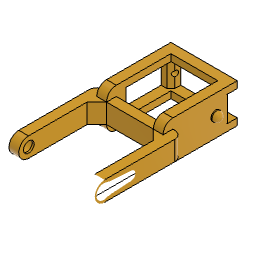
crane assembly v14 (Autodesk Fusion 360 archive; units mm, degrees)
design "link"
Autodesk Fusion 360 part; units mm, degrees
note: some values were not read from the file. Chosen so that the rebuilt part matches the saved one: which bodies a step acts on; which face or edge a step refers to. Set by a fixed rule: which sketch regions a step uses.
sketch "Sketch1" plane through (0, 0, 0) normal (1, 0, 0) x (0, 1, 0)
  line L0 (0, 0) -> (50, 0)
  line L1 (50, 0) -> (50, 10)
  line L2 (50, 10) -> (0, 10)
  line L3 (0, 10) -> (0, 0)
  dimension "d1" = 50
  dimension "d2" = 10
  constraint horizontal L0
  constraint vertical L1
  constraint horizontal L2
  constraint vertical L3
  constraint coincident L0.start L3.end
  measures "d1" distance of L0.start L0.end
  measures "d2" distance of L0.start L2.end
extrude "Extrude1" add sketch "Sketch1" along normal blind 5 makes body 1
sketch "Sketch2" plane through (5, 0, 0) normal (1, 0, 0) x (0, 1, 0)
  line L0 (0, 10) -> (0, 0)
  line L1 (0, 0) -> (50, 0)
  line L2 (50, 0) -> (50, 10)
  line L3 (50, 10) -> (0, 10)
  line L4 (0, 5) -> (4.5, 5) construction
  circle A0 centre (4.5, 5) radius 3.7
  line L5 (4.5, 5) -> (6.5, 5) construction
  line L6 (6.5, 5) -> (6.5, 8.1129)
  line L7 (6.5, 5) -> (6.5, 1.8871)
  line L8 (4.5, 5) -> (18.5, 5) construction
  circle A1 centre (18.5, 5) radius 2.25
  line L9 (18.5, 5) -> (18.5, 7.25) construction
  line L10 (18.5, 5) -> (18.5, 2.75) construction
  line L11 (6.5, 1.8871) -> (18.5, 2.75)
  line L12 (6.5, 8.1129) -> (18.5, 7.25)
  dimension "d5" = 4.5
  dimension "d6" = 7.4
  dimension "d11" = 2
  dimension "d12" = 14
  dimension "d13" = 4.5
  constraint midpoint L0 L4.start
  constraint perpendicular L0 L4
  constraint coincident L4.end A0.centre
  constraint parallel L4 L5
  constraint coincident A0 L6.end
  constraint perpendicular L5 L6
  constraint coincident A0 L7.end
  constraint perpendicular L5 L7
  constraint parallel L5 L8
  constraint coincident L8.end A1.centre
  constraint coincident A1 L9.end
  constraint perpendicular L8 L9
  constraint coincident A1 L10.end
  constraint perpendicular L8 L10
  measures "d5" distance of L4.start L4.end
  measures "d6" diameter of A0
  measures "d11" distance of L4.end L5.end
  measures "d12" distance of L4.end L8.end
  measures "d13" diameter of A1
extrude "Extrude2" cut sketch "Sketch2" against normal blind 5 contours A0 L6 L7 | A0 L6 L7 bodies 1
fillet "Fillet1" radius 5 2 edges at (2.5, 0, 10) (2.5, 0, 0) on bodies 1
extrude "Extrude3" cut sketch "Sketch2" against normal blind 3 contours A0 A1 L11 L12 | A1 bodies 1
fillet "Fillet2" radius 10 2 edges at (3.5, 6.5, 8.1129) (3.5, 6.5, 1.8871) on bodies 1
sketch "Sketch3" plane through (0, 0, 0) normal (-1, 0, 0) x (0, -1, 0)
  circle A0 centre (-4.5, 5) radius 3.7
  arc A1 (-5, 0) -> (-5, 10) centre (-5, 5) ccw
  line L0 (-5, 10) -> (-50, 10)
  line L1 (-50, 10) -> (-50, 0)
  line L2 (-50, 0) -> (-5, 0)
  line L3 (-50, 10) -> (-40, 10) construction
  line L4 (-40, 10) -> (-40, 0) construction
  line L5 (-40, 0) -> (-50, 0) construction
  line L6 (-50, 0) -> (-50, 10) construction
  line L7 (-40, 10) -> (-45, 10)
  line L8 (-45, 10) -> (-45, 0)
  line L9 (-45, 0) -> (-40, 0)
  line L10 (-40, 0) -> (-40, 10)
  dimension "d18" = 10
  dimension "d19" = 5
  constraint horizontal L3
  constraint vertical L4
  constraint horizontal L5
  constraint vertical L6
  constraint coincident L0.end L1.start
  constraint horizontal L7
  constraint vertical L8
  constraint horizontal L9
  constraint vertical L10
  measures "d18" distance of L0.end L3.end
  measures "d19" distance of L3.end L7.end
extrude "Extrude4" add sketch "Sketch3" along normal blind 39 contours L0 L2 L7 L8 L9 L10 bodies 1
sketch "Sketch4" plane through (0, 40, 0) normal (0, -1, 0) x (1, 0, 0)
  line L0 (0, 0) -> (0, 10)
  line L1 (0, 10) -> (-39, 10)
  line L2 (-39, 10) -> (-39, 0)
  line L3 (-39, 0) -> (0, 0)
  line L4 (-39, 10) -> (-34, 10)
  line L5 (-34, 10) -> (-34, 0)
  line L6 (-34, 0) -> (-39, 0)
  line L7 (-39, 0) -> (-39, 10)
  dimension "d22" = 5
  constraint horizontal L4
  constraint vertical L5
  constraint horizontal L6
  constraint vertical L7
  constraint coincident L1.end L2.start
  measures "d22" distance of L1.end L4.end
extrude "Extrude5" add sketch "Sketch4" along normal blind 40 contours L1 L2 L3 L4 L5 L6 L7 bodies 1
sketch "Sketch5" plane through (-34, 0, 0) normal (1, 0, 0) x (0, 1, 0)
  line L0 (40, 0) -> (40, 10)
  line L1 (40, 10) -> (0, 10)
  line L2 (0, 10) -> (0, 0)
  line L3 (0, 0) -> (40, 0)
  line L4 (0, 5) -> (5.175, 5) construction
  circle A0 centre (5.175, 5) radius 2.75
  dimension "d25" = 5.175
  dimension "d26" = 5.5
  constraint midpoint L2 L4.start
  constraint perpendicular L2 L4
  constraint coincident L4.end A0.centre
  measures "d25" distance of L4.start L4.end
  measures "d26" diameter of A0
extrude "Extrude6" cut sketch "Sketch5" against normal blind 3 contours A0 bodies 1
fillet "Fillet3" radius 2 1 edges at (-37, 2.6111, 5.9944) on bodies 1
fillet "Fillet4" radius 5 2 edges at (-36.5, 0, 10) (-36.5, 0, 0) on bodies 1
sketch "Sketch6" plane through (0, 0, 0) normal (0, 0, -1) x (1, 0, 0)
  line L0 (0, -40) -> (-34, -40)
  line L1 (-34, -40) -> (-34, -5)
  line L2 (-34, -5) -> (-39, -5)
  line L3 (-39, -5) -> (-39, -45)
  line L4 (-39, -45) -> (0, -45)
  line L5 (0, -40) -> (5, -40)
  line L6 (5, -40) -> (5, -35)
  line L7 (5, -35) -> (0, -35)
  line L8 (0, -35) -> (0, -40)
  line L9 (0, -45) -> (0, -50)
  line L10 (0, -50) -> (5, -50)
  line L11 (5, -50) -> (5, -5)
  line L12 (5, -5) -> (0, -5)
  line L13 (0, -5) -> (0, -40)
  line L14 (5, -50) -> (0, -50)
  line L15 (0, -50) -> (0, -45)
  line L16 (0, -45) -> (5, -45)
  line L17 (5, -45) -> (5, -50)
  dimension "d35" = 5
  constraint horizontal L5
  constraint vertical L6
  constraint horizontal L7
  constraint vertical L8
  constraint horizontal L14
  constraint vertical L15
  constraint horizontal L16
  constraint vertical L17
  constraint coincident L4.end L9.start
  constraint coincident L10.end L11.start
  measures "d35" distance of L0.start L7.end
extrude "Extrude8" add sketch "Sketch6" along normal blind 5 contours L9 L10 L11 L14 L15 L16 L17 bodies 1
sketch "Sketch7" plane through (0, 0, 10) normal (0, 0, 1) x (-1, 0, 0)
  line L0 (0, -45) -> (39, -45)
  line L1 (39, -45) -> (39, -5)
  line L2 (39, -5) -> (34, -5)
  line L3 (34, -5) -> (34, -40)
  line L4 (34, -40) -> (0, -40)
  line L5 (0, -40) -> (-5, -40)
  line L6 (-5, -40) -> (-5, -35)
  line L7 (-5, -35) -> (0, -35)
  line L8 (0, -35) -> (0, -40)
  line L9 (0, -40) -> (0, -5)
  line L10 (0, -5) -> (-5, -5)
  line L11 (-5, -5) -> (-5, -50)
  line L12 (-5, -50) -> (0, -50)
  line L13 (0, -50) -> (0, -45)
  line L14 (0, -50) -> (-5, -50)
  line L15 (-5, -50) -> (-5, -45)
  line L16 (-5, -45) -> (0, -45)
  line L17 (0, -45) -> (0, -50)
  dimension "d38" = 5
  dimension "d93" = 5
  constraint horizontal L5
  constraint vertical L6
  constraint horizontal L7
  constraint vertical L8
  constraint horizontal L14
  constraint vertical L15
  constraint horizontal L16
  constraint vertical L17
  constraint coincident L12.end L13.start
  measures "d38" distance of L4.end L7.end
  measures "d93" distance of L12.end L0.start
extrude "Extrude9" add sketch "Sketch7" along normal blind 5 contours L11 L12 L13 L14 L15 L16 L17 bodies 1
sketch "Sketch8" plane through (0, 45, 0) normal (0, 1, 0) x (-1, 0, 0)
  line L0 (0, 0) -> (39, 0)
  line L1 (39, 0) -> (39, 10)
  line L2 (39, 10) -> (0, 10)
  line L3 (39, 0) -> (34, 0)
  line L4 (34, 0) -> (34, 15)
  line L5 (34, 15) -> (39, 15)
  line L6 (39, 15) -> (39, 0)
  line L7 (39, 0) -> (34, 0)
  line L8 (34, 0) -> (34, -5)
  line L9 (34, -5) -> (39, -5)
  line L10 (39, -5) -> (39, 0)
  line L11 (0, 10) -> (0, 0)
  dimension "d41" = 5
  dimension "d42" = 15
  dimension "d43" = 5
  dimension "d44" = 5
  constraint horizontal L3
  constraint vertical L4
  constraint horizontal L5
  constraint vertical L6
  constraint coincident L0.end L1.start
  constraint horizontal L7
  constraint vertical L8
  constraint horizontal L9
  constraint vertical L10
  measures "d41" distance of L0.end L3.end
  measures "d42" distance of L0.end L5.end
  measures "d43" distance of L0.end L3.end
  measures "d44" distance of L0.end L9.end
extrude "Extrude10" add sketch "Sketch8" along normal blind 5 contours L0 L1 L2 L3 L4 L6 L7 | L0 L3 L7 L8 L9 L10 | L2 L4 L5 L6 bodies 1
split "Split1" by plane through (0, 45, 10) normal (0, 1, 0) bodies 1 makes body 2 at (-34, 48.3333, 3.3333) makes body 3 at (0, 48.3333, 3.3333)
move_body "Move1" bodies 2 to x (1, 0, 0) y (0, 1, 0) z (0, 0, 1) at (5, 0, 0)
move_body "Move3" bodies 3 to x (1, 0, 0) y (0, 1, 0) z (0, 0, 1) at (-5, 0, 0)
chamfer "Chamfer4" distance 5 angle 45 2 edges at (-34, 40, 5) (0, 40, 5) on bodies 1
combine "Combine1" operation add target body 1 tool bodies 3 2
revolve "Revolve1" add 2 faces at (-3.3333, 45, -1.6667) (-30.6667, 45, -1.6667) angle 360 about axis through (-29, 45, 0) along (1, 0, 0) on bodies 1 bodies 1
revolve "Revolve2" add 2 faces at (-30.6667, 45, 13.3333) (-1.6667, 45, 11.6667) angle 360 about axis through (-5, 45, 10) along (-1, 0, 0) on bodies 1 bodies 1
sketch "Sketch16" plane through (0, 50, 0) normal (0, 1, 0) x (-1, 0, 0)
  line L0 (29, 15) -> (29, -5)
  line L1 (29, -5) -> (34, -5)
  line L2 (34, -5) -> (34, 15)
  line L3 (34, 15) -> (29, 15)
  line L4 (34, -5) -> (29, -5)
  line L5 (29, -5) -> (29, -1.5)
  line L6 (29, -1.5) -> (34, -1.5)
  line L7 (34, -1.5) -> (34, -5)
  line L8 (34, 15) -> (29, 15)
  line L9 (29, 15) -> (29, 11.5)
  line L10 (29, 11.5) -> (34, 11.5)
  line L11 (34, 11.5) -> (34, 15)
  dimension "d96" = 3.5
  dimension "d97" = 3.5
  constraint horizontal L4
  constraint vertical L5
  constraint horizontal L6
  constraint vertical L7
  constraint coincident L1.end L2.start
  constraint horizontal L8
  constraint vertical L9
  constraint horizontal L10
  constraint vertical L11
  constraint coincident L2.end L3.start
  measures "d96" distance of L1.end L6.end
  measures "d97" distance of L2.end L10.end
extrude "Extrude12" add sketch "Sketch16" along normal blind 28 contours L0 L2 L3 L8 L9 L10 L11 | L0 L1 L2 L4 L5 L6 L7 bodies 1
sketch "Sketch17" plane through (0, 0, 11.5) normal (0, 0, -1) x (1, 0, 0)
  line L0 (-29, -50) -> (-34, -50)
  line L1 (-34, -50) -> (-34, -78)
  line L2 (-34, -78) -> (-29, -78)
  line L3 (-29, -78) -> (-29, -50)
  line L4 (-34, -78) -> (-29, -78)
  line L5 (-29, -78) -> (-29, -73)
  line L6 (-29, -73) -> (-34, -73)
  line L7 (-34, -73) -> (-34, -78)
  dimension "d98" = 5
  constraint horizontal L4
  constraint vertical L5
  constraint horizontal L6
  constraint vertical L7
  constraint coincident L1.end L2.start
  measures "d98" distance of L1.end L6.end
extrude "Extrude13" add sketch "Sketch17" along normal blind 13 contours L1 L2 L3 L4 L5 L6 L7 bodies 1
sketch "Sketch12" plane through (-39, 0, 0) normal (-1, 0, 0) x (0, -1, 0)
  line L0 (-73, 5) -> (-75.5, 5) construction
  circle A0 centre (-75.5, 5) radius 1.4
  line L1 (-45, 10) -> (-45, 0)
  line L2 (-45, 0) -> (-5, 0)
  arc A1 (-5, 0) -> (-5, 10) centre (-5, 5) ccw
  line L3 (-5, 10) -> (-45, 10)
  dimension "d64" = 2.5
  dimension "d65" = 2.8
  constraint coincident L0.end A0.centre
  measures "d64" distance of L0.start L0.end
  measures "d65" diameter of A0
extrude "Extrude14" cut sketch "Sketch12" against normal blind 10 contours A0 bodies 1
extrude "Extrude15" add 1 faces at (-1.6667, 50, 1.6667) along direction (0, 1, 0) blind 28 on bodies 1 bodies 1
sketch "Sketch18" plane through (-29, 0, 0) normal (1, 0, 0) x (0, 1, 0)
  circle A0 centre (75.5, 5) radius 1.4
  line L0 (73, -1.5) -> (50, -1.5)
  line L1 (50, -1.5) -> (50, 11.5)
  line L2 (50, 11.5) -> (73, 11.5)
  line L3 (73, 11.5) -> (73, -1.5)
  line L4 (78, -5) -> (78, 15)
  line L5 (78, 15) -> (45, 15)
  arc A1 (45, 15) -> (40, 10) centre (45, 10) ccw
  line L6 (40, 10) -> (45, 10)
  line L7 (45, 10) -> (45, 0)
  line L8 (45, 0) -> (40, 0)
  arc A2 (40, 0) -> (45, -5) centre (45, 0) ccw
  line L9 (45, -5) -> (78, -5)
  line L10 (78, 15) -> (73, 15)
  line L11 (73, 15) -> (73, 11.5)
  line L12 (73, 11.5) -> (78, 11.5)
  line L13 (78, 11.5) -> (78, 15)
  line L14 (78, -5) -> (73, -5)
  line L15 (73, -5) -> (73, -1.5)
  line L16 (73, -1.5) -> (78, -1.5)
  line L17 (78, -1.5) -> (78, -5)
  constraint horizontal L10
  constraint vertical L11
  constraint horizontal L12
  constraint vertical L13
  constraint coincident L2.end L3.start
  constraint coincident L4.end L5.start
  constraint horizontal L14
  constraint vertical L15
  constraint horizontal L16
  constraint vertical L17
  constraint coincident L0.start L3.end
  constraint coincident L4.start L9.end
extrude "Extrude16" add sketch "Sketch18" along normal blind 24 contours L4 L9 L14 L15 L16 L17 | L4 L5 L10 L11 L12 L13 bodies 1
sketch "Sketch14" plane through (0, 0, 0) normal (1, 0, 0) x (0, 1, 0)
  line L0 (78, -5) -> (78, 15)
  line L1 (78, 15) -> (78, 11.5) construction
  line L2 (78, 11.5) -> (73, 11.5)
  line L3 (73, 11.5) -> (73, -1.5)
  line L4 (73, -1.5) -> (78, -1.5)
  line L5 (78, -1.5) -> (78, 11.5)
  line L6 (40, 10) -> (45, 10)
  line L7 (45, 10) -> (45, 0)
  line L8 (45, 0) -> (40, 0)
  line L9 (40, 0) -> (40, 10)
  arc A0 (40, 0) -> (45, -5) centre (45, 0) ccw
  line L10 (45, 10) -> (45, 0)
  line L11 (45, 0) -> (40, 0)
  line L12 (45, -5) -> (78, -5)
  line L13 (78, 15) -> (45, 15)
  arc A1 (45, 15) -> (40, 10) centre (45, 10) ccw
  line L14 (40, 10) -> (45, 10)
  point P0 (40, 0)
  point P1 (40, 0)
  dimension "d75" = 3.5
  dimension "d76" = 5
  dimension "d77" = 13
  dimension "d80" = 5
  dimension "d81" = 10
  constraint coincident L0.end L1.start
  constraint horizontal L2
  constraint vertical L3
  constraint horizontal L4
  constraint vertical L5
  constraint horizontal L6
  constraint vertical L7
  constraint horizontal L8
  constraint vertical L9
  measures "d75" distance of L0.end L1.end
  measures "d76" distance of L1.end L2.end
  measures "d77" distance of L1.end L4.end
  measures "d80" distance of L6.start L6.end
  measures "d81" distance of L6.start P1
extrude "Extrude17" cut sketch "Sketch14" against normal blind 5 contours L0 L2 L3 L4 L5 | L6 L7 L8 L9 L10 L11 L14 bodies 1
sketch "Sketch15" plane through (0, 0, 0) normal (1, 0, 0) x (0, 1, 0)
  line L0 (78, 11.5) -> (78, 15)
  line L1 (73, -1.5) -> (73, 11.5)
  line L2 (73, 11.5) -> (78, 11.5)
  line L3 (73, 5) -> (67, 5) construction
  circle A0 centre (67, 5) radius 2.5
  arc A1 (40, 0) -> (45, -5) centre (45, 0) ccw
  line L4 (78, -1.5) -> (73, -1.5)
  line L5 (78, 15) -> (45, 15)
  arc A2 (45, 15) -> (40, 10) centre (45, 10) ccw
  line L6 (40, 10) -> (45, 10)
  line L7 (45, 10) -> (45, 0)
  line L8 (45, 0) -> (40, 0)
  line L9 (45, -5) -> (78, -5)
  line L10 (78, -5) -> (78, -1.5)
  dimension "d84" = 6
  dimension "d85" = 5
  constraint midpoint L1 L3.start
  constraint coincident L3.end A0.centre
  measures "d84" distance of L3.start L3.end
  measures "d85" diameter of A0
extrude "Extrude18" add sketch "Sketch15" along normal blind 3 contours A0 bodies 1
fillet "Fillet7" radius 2.5 1 edges at (3, 64.6692, 4.096) on bodies 1
chamfer "Chamfer2" distance 5 angle 45 1 edges at (-5, 73, 5) on bodies 1
chamfer "Chamfer5" distance 2 angle 45 1 edges at (-29, 73, 5) on bodies 1
sketch "Sketch19" plane through (-29, 0, 0) normal (1, 0, 0) x (0, 1, 0)
  line L0 (73, 11.5) -> (73, 15)
  line L1 (73, 15) -> (45, 15)
  arc A0 (45, 15) -> (40, 10) centre (45, 10) ccw
  line L2 (40, 10) -> (45, 10)
  line L3 (45, 10) -> (45, 0)
  line L4 (45, 0) -> (40, 0)
  arc A1 (40, 0) -> (45, -5) centre (45, 0) ccw
  line L5 (45, -5) -> (73, -5)
  line L6 (73, -5) -> (73, -1.5)
  line L7 (73, -1.5) -> (50, -1.5)
  line L8 (50, -1.5) -> (50, 11.5)
  line L9 (50, 11.5) -> (73, 11.5)
  line L10 (45, 5) -> (47.5, 5)
  circle A2 centre (47.5, 5) radius 1.4
  dimension "d100" = 2.5
  dimension "d101" = 2.8
  constraint midpoint L3 L10.start
  constraint perpendicular L8 L10
  constraint coincident L10.end A2.centre
  measures "d100" distance of L10.start L10.end
  measures "d101" diameter of A2
extrude "Extrude19" cut sketch "Sketch19" against normal blind 5 contours A2 bodies 1
fillet "Fillet8" radius 4 2 edges at (-39, 45, 5) (5, 45, 5) on bodies 1

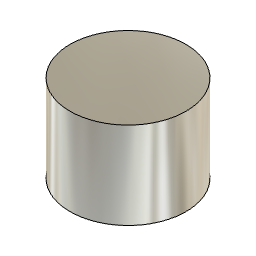
design "electromagnet"
Autodesk Fusion 360 part; units mm, degrees
sketch "Sketch1" plane through (0, 0, 0) normal (0, 0, 1) x (1, 0, 0)
  circle A0 centre (0, 0) radius 10
  dimension "d1" = 20
  constraint coincident A0.centre origin
  measures "d1" diameter of A0
extrude "Extrude1" add sketch "Sketch1" along normal blind 15
sketch "Sketch2" plane through (0, 0, 0) normal (0, 0, -1) x (1, 0, 0)
  circle A0 centre (0, 0) radius 10
  circle A1 centre (0, 0) radius 2
  dimension "d4" = 4
  constraint concentric A0 A1
  measures "d4" diameter of A1
extrude "Extrude2" cut sketch "Sketch2" against normal blind 5 contours A1

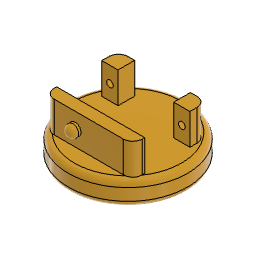
design "first crane stand"
part number: Configuration 1
Autodesk Fusion 360 part; units mm, degrees
sketch "Sketch1" plane through (0, 0, 0) normal (0, 0, 1) x (1, 0, 0)
  circle A0 centre (0, 0) radius 25
  dimension "d1" = 50
  constraint coincident A0.centre origin
  measures "d1" diameter of A0
extrude "Extrude1" add sketch "Sketch1" along normal blind 10
sketch "Sketch2" plane through (0, 0, 0) normal (0, 0, -1) x (1, 0, 0)
  circle A0 centre (0, 0) radius 25
  line L0 (0, 0) -> (0, -10) construction
  circle A1 centre (0, -10) radius 3.5
  line L1 (0, -10) -> (0, -7.737) construction
  line L2 (0, -7.737) -> (-2.67, -7.737) construction
  line L3 (0, -7.737) -> (2.67, -7.737) construction
  line L4 (0, -10) -> (0, 3.98) construction
  circle A2 centre (0, 3.98) radius 2.1005
  line L5 (2.67, -7.737) -> (2.098, 4.0815)
  line L6 (-2.67, -7.737) -> (-2.098, 4.0815)
  dimension "d4" = 10
  dimension "d5" = 7
  dimension "d6" = 2.263
  dimension "d7" = 13.98
  dimension "d8" = 4.201
  constraint coincident A0.centre L0.start
  constraint vertical L0
  constraint coincident L0.end A1.centre
  constraint parallel L0 L1
  constraint coincident A1 L2.end
  constraint perpendicular L0 L2
  constraint coincident A1 L3.end
  constraint perpendicular L1 L3
  constraint parallel L0 L4
  constraint coincident L4.end A2.centre
  constraint coincident A2 L5.end
  constraint tangent A2 L5
  constraint coincident A2 L6.end
  constraint tangent A2 L6
  measures "d4" distance of A0.centre L0.end
  measures "d5" diameter of A1
  measures "d6" distance of L0.end L1.end
  measures "d7" distance of L0.end L4.end
  measures "d8" diameter of A2
extrude "Extrude2" cut sketch "Sketch2" against normal blind 2 contours A1 | A1 A2 L5 L6 | A2
sketch "Sketch14" plane through (0, 0, 10) normal (0, 0, 1) x (-1, 0, 0)
  circle A0 centre (0, 0) radius 25
  line L0 (18.5, 11.5) -> (-18.5, 11.5) construction
  line L1 (-18.5, 11.5) -> (-18.5, -11.5) construction
  line L2 (-18.5, -11.5) -> (18.5, -11.5) construction
  line L3 (18.5, -11.5) -> (18.5, 11.5) construction
  line L4 (18.5, 11.5) -> (-18.5, -11.5) construction
  line L5 (-18.5, 11.5) -> (18.5, -11.5) construction
  line L6 (-18.5, -11.5) -> (-11.7, -11.5)
  line L7 (-11.7, -11.5) -> (-11.7, -7.5)
  line L8 (-11.7, -7.5) -> (-18.5, -7.5)
  line L9 (-18.5, -7.5) -> (-18.5, -11.5)
  line L10 (18.5, -11.5) -> (11.7, -11.5)
  line L11 (11.7, -11.5) -> (11.7, -7.5)
  line L12 (11.7, -7.5) -> (18.5, -7.5)
  line L13 (18.5, -7.5) -> (18.5, -11.5)
  line L14 (18.5, 11.5) -> (-18.5, 11.5)
  line L15 (-18.5, 11.5) -> (-18.5, 16.5)
  line L16 (-18.5, 16.5) -> (18.5, 16.5)
  line L17 (18.5, 16.5) -> (18.5, 11.5)
  dimension "d95" = 37
  dimension "d96" = 23
  dimension "d97" = 6.8
  dimension "d98" = 4
  dimension "d99" = 6.8
  dimension "d100" = 4
  dimension "d101" = 37
  dimension "d102" = 5
  constraint horizontal L0
  constraint perpendicular L0 L1
  constraint parallel L0 L2
  constraint parallel L1 L3
  constraint coincident L4 A0.centre
  constraint coincident L5 A0.centre
  constraint coincident A0.centre origin
  constraint horizontal L6
  constraint vertical L7
  constraint horizontal L8
  constraint vertical L9
  constraint horizontal L10
  constraint vertical L11
  constraint horizontal L12
  constraint vertical L13
  constraint horizontal L14
  constraint vertical L15
  constraint horizontal L16
  constraint vertical L17
  measures "d95" distance of L1.end L2.end
  measures "d96" distance of L0.end L1.end
  measures "d97" distance of L1.end L6.end
  measures "d98" distance of L1.end L8.end
  measures "d99" distance of L2.end L10.end
  measures "d100" distance of L2.end L12.end
  measures "d101" distance of L0.start L0.end
  measures "d102" distance of L0.start L16.end
extrude "Extrude15" add sketch "Sketch14" along normal blind 13 contours L6 L7 L8 L9 | L10 L11 L12 L13 | L14 L15 L16 L17
sketch "Sketch15" plane through (0, 11.5, 0) normal (0, 1, 0) x (-1, 0, 0)
  line L0 (-18.5, 10) -> (-11.7, 10)
  line L1 (-11.7, 10) -> (-11.7, 23)
  line L2 (-11.7, 23) -> (-18.5, 23)
  line L3 (-18.5, 23) -> (-18.5, 10)
  line L4 (-15.1, 10) -> (-15.1, 16.25) construction
  circle A0 centre (-15.1, 16.25) radius 1.4
  dimension "d105" = 6.25
  dimension "d106" = 2.8
  constraint midpoint L0 L4.start
  constraint perpendicular L0 L4
  constraint coincident L4.end A0.centre
  measures "d105" distance of L4.start L4.end
  measures "d106" diameter of A0
sketch "Sketch16" plane through (0, 11.5, 0) normal (0, 1, 0) x (-1, 0, 0)
  line L0 (11.7, 10) -> (18.5, 10)
  line L1 (18.5, 10) -> (18.5, 23)
  line L2 (18.5, 23) -> (11.7, 23)
  line L3 (11.7, 23) -> (11.7, 10)
  line L4 (15.1, 10) -> (15.1, 16.25) construction
  circle A0 centre (15.1, 16.25) radius 1.4
  dimension "d107" = 6.25
  dimension "d108" = 2.8
  constraint midpoint L0 L4.start
  constraint perpendicular L0 L4
  constraint coincident L4.end A0.centre
  measures "d107" distance of L4.start L4.end
  measures "d108" diameter of A0
extrude "Extrude16" cut sketch "Sketch16" sketch "Sketch15" against normal blind 4.475 contours A0 of sketch 2 contours A0
sketch "Sketch17" plane through (0, -16.5, 0) normal (0, -1, 0) x (1, 0, 0)
  line L0 (-18.5, 10) -> (18.5, 10)
  line L1 (18.5, 10) -> (18.5, 23)
  line L2 (18.5, 23) -> (-18.5, 23)
  line L3 (-18.5, 23) -> (-18.5, 10)
  line L4 (-18.5, 10) -> (18.5, 23) construction
  line L5 (18.5, 10) -> (-18.5, 23) construction
  line L6 (0, 16.5) -> (-5.7, 16.5) construction
  circle A0 centre (-5.7, 16.5) radius 2.5
  dimension "d120" = 5.7
  dimension "d121" = 5
  constraint coincident L0.start L3.end
  constraint coincident L1.end L2.start
  constraint coincident L0.end L1.start
  constraint coincident L2.end L3.start
  constraint horizontal L6
  constraint coincident L6.end A0.centre
  measures "d120" distance of L6.start L6.end
  measures "d121" diameter of A0
extrude "Extrude17" add sketch "Sketch17" along normal blind 3.5 contours A0
extrude "Extrude18" add 2 faces at (15.0651, 11.5, 21.2154) (-15.0651, 11.5, 21.2154) along direction (0, 1, 0) blind 3
fillet "Fillet8" radius 2.5 1 faces at (-6.4508, -20, 16.1384)
fillet "Fillet9" radius 4 2 edges at (18.5, -16.5, 16.5) (-18.5, -16.5, 16.5)
fillet "Fillet10" radius 2.5 2 edges at (-23.3082, -9.0404, 10) (-23.3082, -9.0404, 0)
fillet "Fillet11" radius 4 2 edges at (-18.5, 14.5, 16.3945) (18.5, 14.5, 16.3945)
equation "fullServoLength = 32.45 mm"

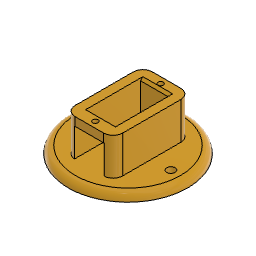
design "crane_base"
Autodesk Fusion 360 part; units mm, degrees
sketch "Sketch1" plane through (0, 0, 0) normal (0, 0, 1) x (1, 0, 0)
  circle A0 centre (0, 0) radius 25
  line L0 (0, 0) -> (-18, 0) construction
  line L1 (0, 0) -> (18, 0) construction
  circle A1 centre (-18, 0) radius 1.75
  circle A2 centre (18, 0) radius 1.75
  dimension "d1" = 50
  dimension "d25" = 18
  dimension "d26" = 18
  dimension "d27" = 3.5
  dimension "d28" = 3.5
  constraint coincident A0.centre L0.start
  constraint horizontal L0
  constraint parallel L0 L1
  constraint coincident L0.end A1.centre
  constraint coincident L1.end A2.centre
  measures "d1" diameter of A0
  measures "d25" distance of A0.centre L0.end
  measures "d26" distance of A0.centre L1.end
  measures "d27" diameter of A1
  measures "d28" diameter of A2
extrude "Extrude1" add sketch "Sketch1" along normal blind 3
sketch "Sketch2" plane through (0, 0, 3) normal (0, 0, 1) x (-1, 0, 0)
  circle A0 centre (0, 0) radius 25
  line L0 (-6.25, 11.5) -> (6.25, 11.5)
  line L1 (6.25, 11.5) -> (6.25, -11.5)
  line L2 (6.25, -11.5) -> (-6.25, -11.5)
  line L3 (-6.25, -11.5) -> (-6.25, 11.5)
  line L4 (-6.25, 11.5) -> (6.25, -11.5) construction
  line L5 (6.25, 11.5) -> (-6.25, -11.5) construction
  line L6 (-10, -16.225) -> (10, -16.225)
  line L7 (10, -16.225) -> (10, 16.225)
  line L8 (10, 16.225) -> (-10, 16.225)
  line L9 (-10, 16.225) -> (-10, -16.225)
  line L10 (-10, -16.225) -> (10, 16.225) construction
  line L11 (10, -16.225) -> (-10, 16.225) construction
  circle A1 centre (-18, 0) radius 1.75
  circle A2 centre (18, 0) radius 1.75
  dimension "d4" = 12.5
  dimension "d5" = 23
  dimension "d6" = 20
  dimension "d7" = 32.45
  constraint horizontal L0
  constraint perpendicular L0 L1
  constraint parallel L0 L2
  constraint parallel L1 L3
  constraint coincident L4 A0.centre
  constraint coincident L5 A0.centre
  constraint coincident A0.centre origin
  constraint horizontal L6
  constraint perpendicular L6 L7
  constraint parallel L6 L8
  constraint parallel L7 L9
  constraint coincident L10 A0.centre
  constraint coincident L11 A0.centre
  measures "d4" distance of L1.end L2.end
  measures "d5" distance of L0.end L1.end
  measures "d6" distance of L7.end L8.end
  measures "d7" distance of L6.end L7.end
extrude "Extrude2" add sketch "Sketch2" along normal blind 15.55 contours L6 L7 L8 L9
sketch "Sketch3" plane through (0, 0, 18.55) normal (0, 0, 1) x (-1, 0, 0)
  line L0 (6.25, -11.5) -> (-6.25, -11.5)
  line L1 (-6.25, -11.5) -> (-6.25, 11.5)
  line L2 (-6.25, 11.5) -> (6.25, 11.5)
  line L3 (6.25, 11.5) -> (6.25, -11.5)
  line L4 (-10, 16.225) -> (-10, -16.225)
  line L5 (-10, -16.225) -> (10, -16.225)
  line L6 (10, -16.225) -> (10, 16.225)
  line L7 (10, 16.225) -> (-10, 16.225)
  line L8 (0, 16.225) -> (0, 13.667) construction
  line L9 (0, -16.225) -> (0, -13.667) construction
  circle A0 centre (0, -13.667) radius 1.1
  circle A1 centre (0, 13.667) radius 1.1
  dimension "d10" = 2.558
  dimension "d11" = 2.558
  dimension "d12" = 2.2
  dimension "d13" = 2.2
  constraint midpoint L7 L8.start
  constraint perpendicular L7 L8
  constraint midpoint L5 L9.start
  constraint perpendicular L5 L9
  constraint coincident L9.end A0.centre
  constraint coincident L8.end A1.centre
  measures "d10" distance of L8.start L8.end
  measures "d11" distance of L9.start L9.end
  measures "d12" diameter of A0
  measures "d13" diameter of A1
extrude "Extrude3" cut sketch "Sketch3" against normal blind 10 contours A0 | A1
sketch "Sketch4" plane through (0, -16.225, 0) normal (0, -1, 0) x (1, 0, 0)
  line L0 (-10, 3) -> (10, 3)
  line L1 (10, 3) -> (10, 18.55)
  line L2 (10, 18.55) -> (-10, 18.55)
  line L3 (-10, 18.55) -> (-10, 3)
  line L4 (0, 3) -> (-6.25, 3) construction
  line L5 (-6.25, 3) -> (6.25, 3)
  line L6 (6.25, 3) -> (6.25, 15)
  line L7 (6.25, 15) -> (-6.25, 15)
  line L8 (-6.25, 15) -> (-6.25, 3)
  dimension "d16" = 6.25
  dimension "d17" = 12.5
  dimension "d18" = 12
  constraint midpoint L0 L4.start
  constraint parallel L0 L4
  constraint horizontal L5
  constraint vertical L6
  constraint horizontal L7
  constraint vertical L8
  measures "d16" distance of L4.start L4.end
  measures "d17" distance of L4.end L5.end
  measures "d18" distance of L4.end L7.end
extrude "Extrude4" cut sketch "Sketch4" against normal blind 4.725 contours L0 L5 L6 L7 L8
fillet "Fillet2" radius 4 4 edges at (10, -16.225, 10.775) (10, 16.225, 10.775) (-10, 16.225, 10.775) (-10, -16.225, 10.775)
fillet "Fillet3" radius 3 1 edges at (-23.3082, -9.0404, 3)
chamfer "Chamfer1" distance 2 angle 45 1 edges at (0, -11.5, 15)
chamfer "Chamfer2" distance 1 angle 45 1 edges at (0, 11.5, 18.55)

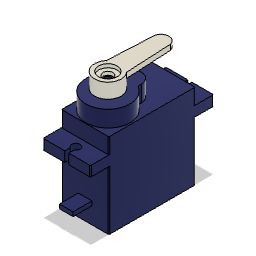
design "SG90 9g servo"
Autodesk Fusion 360 part; units mm, degrees
sketch "Body" plane through (0, 0, 0) normal (0, 1, 0) x (1, 0, 0) in component "servo"
  line L0 (6.25, -11.375) -> (-6.25, -11.375)
  line L1 (-6.25, -11.375) -> (-6.25, 11.375)
  line L2 (-6.25, 11.375) -> (6.25, 11.375)
  line L3 (6.25, 11.375) -> (6.25, -11.375)
  line L4 (6.25, -11.375) -> (-6.25, 11.375) construction
  line L5 (-6.25, -11.375) -> (6.25, 11.375) construction
  dimension "d6" = 12.5
  dimension "d7" = 22.75
  dimension "d52" = 0
  dimension "d53" = 0
  dimension "d54" = 0
  dimension "d55" = 0
  constraint perpendicular L0 L1
  constraint parallel L0 L2
  constraint parallel L1 L3
  constraint horizontal L0
  constraint coincident L4 origin
  constraint coincident L5 origin
  measures "d6" distance of L1.end L2.end
  measures "d7" distance of L0.end L1.end
extrude "Extrude1" add sketch "Body" along normal blind 22.35 makes body 1 in component "servo"
sketch "Tab" plane through (0, 0, 11.375) normal (0, 0, 1) x (1, 0, 0) in component "servo"
  line L0 (-6.25, 0) -> (6.25, 0)
  line L1 (6.25, 0) -> (6.25, 22.35)
  line L2 (6.25, 22.35) -> (-6.25, 22.35)
  line L3 (-6.25, 22.35) -> (-6.25, 0)
  line L4 (-6.25, 18.2) -> (6.25, 18.2)
  line L5 (6.25, 18.2) -> (6.25, 15.55)
  line L6 (6.25, 15.55) -> (-6.25, 15.55)
  line L7 (-6.25, 15.55) -> (-6.25, 18.2)
  dimension "d10" = 4.15
  dimension "d11" = 2.65
  constraint horizontal L4
  constraint vertical L5
  constraint horizontal L6
  constraint vertical L7
  constraint coincident L1 L5.end
  constraint coincident L3 L4.start
  measures "d10" distance of L1.end L4.end
  measures "d11" distance of L4.end L5.end
extrude "Extrude2" add sketch "Tab" along normal blind 4.85 contours L1 L3 L4 L5 L6 L7 bodies 1 in component "servo"
hole "Hole1" at (0, 18.2, 13.8) direction (0, -1, 0) diameter 2.2 end through all bodies 1 in component "servo"
fillet "Fillet1" radius 0.25 2 edges at (6.25, 16.875, 16.225) (-6.25, 16.875, 16.225) on bodies 1 in component "servo"
sketch "Notch" plane through (0, 0, 16.225) normal (0, 0, 1) x (1, 0, 0) in component "servo"
  line L0 (-6, 18.2) -> (-6, 15.55)
  line L1 (-6, 15.55) -> (6, 15.55)
  line L2 (6, 15.55) -> (6, 18.2)
  line L3 (6, 18.2) -> (-6, 18.2)
  line L4 (-0.525, 18.2) -> (0.525, 18.2)
  line L5 (0.525, 18.2) -> (0.525, 15.55)
  line L6 (0.525, 15.55) -> (-0.525, 15.55)
  line L7 (-0.525, 15.55) -> (-0.525, 18.2)
  dimension "d20" = 1.05
  constraint collinear L3 L4
  constraint collinear L1 L6
  constraint parallel L5 L7
  measures "d20" distance of L4.start L4.end
extrude "Extrude3" cut sketch "Notch" along normal up to surface contours L1 L3 L4 L5 L6 L7 end surface at (0.0548, 17.3167, 14.8986) on bodies 1 bodies 1 in component "servo"
mirror "Mirror1" about plane through (0, 0, 0) normal (0, 0, 1) of "Extrude2", "Hole1", "Fillet1", "Extrude3" in component "servo"
sketch "Bump" plane through (0, 22.35, 0) normal (0, 1, 0) x (-1, 0, 0) in component "servo"
  line L0 (-6.25, -11.375) -> (6.25, -11.375)
  line L1 (6.25, -11.375) -> (6.25, 11.375)
  line L2 (6.25, 11.375) -> (-6.25, 11.375)
  line L3 (-6.25, 11.375) -> (-6.25, -11.375)
  line L4 (-2.8, -0.625) -> (-2.8, 0.2671)
  line L5 (2.8, 0.2671) -> (2.8, -0.625)
  arc A0 (-2.8, -0.625) -> (2.8, -0.625) centre (0, -0.625) ccw
  arc A1 (2.8, 0.2671) -> (-2.8, 0.2671) centre (0, 5.375) ccw
  dimension "d23" = 11.65
  dimension "d24" = 6
  dimension "d25" = 5.6
  dimension "d26" = 6
  dimension "d27" = 6.25
  dimension "d28" = 6.25
  constraint tangent L4 A0
  constraint vertical L4
  constraint tangent L5 A0
  measures "d23" diameter of A1
  measures "d24" distance of L2 A1.centre
  measures "d25" diameter of A0
  measures "d26" distance of A1.centre A0.centre
  measures "d27" distance of L3 A1.centre
  measures "d28" distance of L3 A0.centre
extrude "Extrude4" add sketch "Bump" along normal blind 4.3 contours L4 L5 A0 A1 bodies 1 in component "servo"
fillet "Fillet2" radius 0.25 8 edges at (6.25, 7.775, 11.375) (6.25, 20.275, 11.375) (-6.25, 20.275, 11.375) (-6.25, 7.775, 11.375) (6.25, 7.775, -11.375) (6.25, 20.275, -11.375) (-6.25, 20.275, -11.375) (-6.25, 7.775, -11.375) on bodies 1 in component "servo"
hole "Hole2" at (0, 26.65, 5.375) direction (0, -1, 0) diameter 4.92 depth 15 tip angle 180 bodies 1 in component "servo"
sketch "Wire" plane through (0, 0, 11.375) normal (0, 0, 1) x (1, 0, 0) in component "servo"
  line L0 (-6, 15.55) -> (-6, 0)
  line L1 (-6, 0) -> (6, 0)
  line L2 (6, 0) -> (6, 15.55)
  line L3 (6, 15.55) -> (-6, 15.55)
  line L4 (-1.8, 5.5) -> (1.8, 5.5)
  line L5 (1.8, 5.5) -> (1.8, 4.4)
  line L6 (1.8, 4.4) -> (-1.8, 4.4)
  line L7 (-1.8, 4.4) -> (-1.8, 5.5)
  dimension "d32" = 1.1
  dimension "d33" = 3.6
  dimension "d34" = 5.5
  constraint horizontal L4
  constraint vertical L5
  constraint horizontal L6
  constraint vertical L7
  measures "d32" distance of L4.start L6.end
  measures "d33" distance of L4.start L4.end
  measures "d34" distance of L1 L4.end
extrude "Extrude5" add sketch "Wire" along normal blind 5 contours L4 L5 L6 L7 bodies 1 in component "servo"
cylinder "CylinderPrimitive1" add diameter 4.92 height 2.72 placed x (1, 0, 0) y (0, 0, -1) z (0, 1, 0) at (0, 26.65, 5.375) separate body makes body 2 in component "splined-drive"
extrude "Extrude1'" add 1 faces at (-0.4548, 26.65, 5.9711) along direction (0, -1, 0) blind 15 on bodies 2 bodies 2 in component "splined-drive"
hole "Hole1'" at (0, 29.37, 5.375) direction (0, -1, 0) diameter 1.95 depth 5 tip angle 180 bodies 2 in component "splined-drive"
chamfer "Chamfer1" distance 0.25 angle 45 1 edges at (-2.2935, 29.37, 6.2646) on bodies 2 in component "splined-drive"
sketch "Sketch1" plane through (0, 29.37, 0) normal (0, 1, 0) x (-1, 0, 0) in component "horn"
  circle A0 centre (0, 5.375) radius 3.5
  circle A1 centre (0, 5.375) radius 2.46
  circle A2 centre (0, 5.375) radius 1.31
  dimension "d102" = 0
  dimension "d103" = 0
  dimension "d104" = 0
  dimension "d105" = 0
extrude "Extrude3'" add sketch "Sketch1" against normal blind 2.08 separate body contours A0 makes body 3 in component "horn"
extrude "Extrude6" add 1 faces at (-3.1311, 29.37, 5.0789) along direction (0, 1, 0) blind 1.83 on bodies 3 bodies 3 in component "horn"
extrude "Extrude4'" add sketch "Sketch1" along normal blind 0.9 contours A1 bodies 3 in component "horn"
sketch "Sketch4" plane through (0, 31.2, 0) normal (0, 1, 0) x (-1, 0, 0) in component "horn"
  circle A0 centre (0, 5.375) radius 2.46
  circle A1 centre (0, 5.375) radius 3.5
  line L0 (2.67, 3.112) -> (2.04, -9.105)
  line L1 (-2.67, 3.112) -> (-2.04, -9.105)
  arc A2 (-2.04, -9.105) -> (2.04, -9.105) centre (0, -8.6045) ccw
  constraint coincident A1 L0.start
  constraint coincident A1 L1.start
extrude "Extrude7" add sketch "Sketch4" against normal blind 1.41 contours A1 L0 L1 A2 bodies 3 in component "horn"
component "servo" placed x (1, 0, 0) y (0, 1, 0) z (0, 0, 1) at (0, 0, 0)
component "splined-drive" placed x (1, 0, 0) y (0, 1, 0) z (0, 0, 1) at (0, 0, 0)
component "horn" placed x (1, 0, 0) y (0, 1, 0) z (0, 0, 1) at (0, 0, 0)
